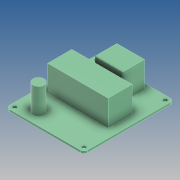
# Autodesk Inventor part: pcb
Saved by Autodesk Inventor 2020 (Build 240168000, 168)
## iProperties
Created: 2021-04-15
Part Number: pcb
Material: Generic
Document SubType Name: Modeling
Designer: stephen
Density: 1 g/cm^3
Appearance: Smooth - Dark Sea Green
Mass: 28.2253 g
Surface Area: 121.709 cm^2
Volume: 28.2253 cm^3
Author: stephen
Autodesk Inventor part; units mm, degrees
ref_plane "YZ Plane" through (0, 0, 0) normal (1, 0, 0) x (0, 1, 0)
ref_plane "XZ Plane" through (0, 0, 0) normal (0, 1, 0) x (-1, 0, 0)
ref_plane "XY Plane" through (0, 0, 0) normal (0, 0, 1) x (1, 0, 0)
sketch "Sketch1" plane through (0, 0, 0) normal (0, 1, 0) x (-1, 0, 0)
  line L0 (-26.035, 33.02) -> (26.035, 33.02)
  line L1 (28.575, 30.48) -> (28.575, -30.48)
  line L2 (26.035, -33.02) -> (-26.035, -33.02)
  line L3 (-28.575, -30.48) -> (-28.575, 30.48)
  line L4 (-28.575, 33.02) -> (28.575, -33.02) construction
  line L5 (28.575, 33.02) -> (-28.575, -33.02) construction
  arc A0 (26.035, -33.02) -> (28.575, -30.48) centre (26.035, -30.48) ccw
  arc A1 (28.575, 30.48) -> (26.035, 33.02) centre (26.035, 30.48) ccw
  arc A2 (-26.035, 33.02) -> (-28.575, 30.48) centre (-26.035, 30.48) ccw
  arc A3 (-28.575, -30.48) -> (-26.035, -33.02) centre (-26.035, -30.48) ccw
  point P0 (0, 0)
  dimension "d0" = 57.15
  dimension "d1" = 66.04
  dimension "d2" = 2.54
  constraints: 12 end point, 8 point on circle, 8 point on line, 8 tangent, 4 centre point, 3 equal radius, 2 midpoint, 2 parallel, 1 horizontal, 1 perpendicular
  measures "d0" distance of L4.start L5.start
  measures "d1" distance of L5.start L4.end
  measures "d2" radius of A0
extrude "Extrusion1" add sketch "Sketch1" along normal blind 1.6
sketch "Sketch2" plane through (0, 1.6, 0) normal (0, 1, 0) x (1, 0, 0)
  line L0 (25.4, -29.845) -> (-25.4, -29.845) construction
  line L1 (-25.4, -29.845) -> (-25.4, 29.845) construction
  line L2 (-25.4, 29.845) -> (25.4, 29.845) construction
  line L3 (25.4, 29.845) -> (25.4, -29.845) construction
  line L4 (25.4, -29.845) -> (-25.4, 29.845) construction
  line L5 (-25.4, -29.845) -> (25.4, 29.845) construction
  circle A0 centre (-25.4, 29.845) radius 1.4605
  circle A1 centre (-25.4, -29.845) radius 1.4605
  circle A2 centre (25.4, -29.845) radius 1.4605
  circle A3 centre (25.4, 29.845) radius 1.4605
  point P0 (0, 0)
  dimension "d5" = 50.8
  dimension "d6" = 59.69
  dimension "d7" = 2.921
  constraints: 12 end point, 4 centre point, 4 coincident, 3 equal radius, 2 midpoint, 2 parallel, 1 horizontal, 1 perpendicular
  measures "d5" distance of L0.start L0.end
  measures "d6" distance of L0.end L1.end
  measures "d7" diameter of A1
extrude "Extrusion2" cut sketch "Sketch2" against normal through all
sketch "Sketch3" plane through (0, 1.6, 0) normal (0, 1, 0) x (1, 0, 0)
  line L0 (-22.225, 8.89) -> (22.225, 8.89)
  line L1 (22.225, 8.89) -> (22.225, -8.89)
  line L2 (22.225, -8.89) -> (-22.225, -8.89)
  line L3 (-22.225, -8.89) -> (-22.225, 8.89)
  line L4 (-22.225, 8.89) -> (22.225, -8.89) construction
  line L5 (22.225, 8.89) -> (-22.225, -8.89) construction
  line L6 (10.9394, 13.1131) -> (-9.3806, 13.1131)
  line L7 (-9.3806, 13.1131) -> (-9.3806, 29.1151)
  line L8 (-9.3806, 29.1151) -> (10.9394, 29.1151)
  line L9 (10.9394, 29.1151) -> (10.9394, 13.1131)
  line L10 (10.9394, 13.1131) -> (-9.3806, 29.1151) construction
  line L11 (-9.3806, 13.1131) -> (10.9394, 29.1151) construction
  circle A0 centre (-13.6746, -24.0899) radius 4.064
  point P0 (0, 0)
  point P1 (0.7794, 21.1141)
  dimension "d10" = 8.128
  dimension "d11" = 17.78
  dimension "d12" = 44.45
  dimension "d13" = 16.002
  dimension "d14" = 20.32
  constraints: 24 end point, 4 midpoint, 4 parallel, 2 horizontal, 2 perpendicular, 1 centre point
  measures "d10" diameter of A0
  measures "d11" distance of L2.end L0.start
  measures "d12" distance of L1.end L2.end
  measures "d13" distance of L6.end L7.end
  measures "d14" distance of L7.end L8.end
extrude "Extrusion3" add sketch "Sketch3" along normal blind 19.05
body "Solid1"
